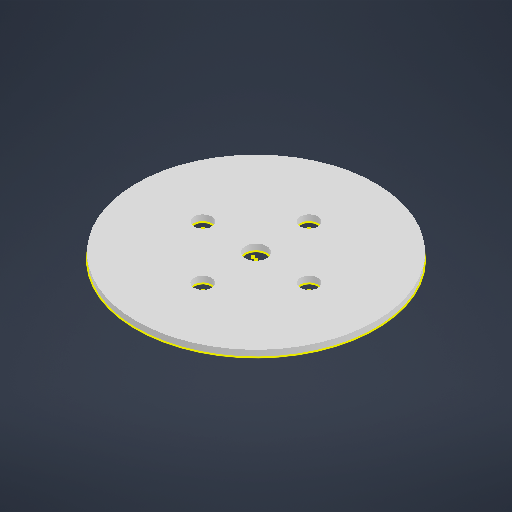
# Autodesk Inventor part: Part5
Saved by Autodesk Inventor 2025.2 (Build 292293000, 293)
## iProperties
Created: 2024-12-26
Part Number: Part5
Material: Generic
Document SubType Name: Sheet Metal
Designer: casey
Density: 1 g/cm^3
Appearance: Default
Flat Pattern Width: 5.715 cm
Flat Pattern Length: 5.715 cm
Flat Pattern Area: 32.6612 cm^2
Sheet Metal Rule: Default
Sheet Metal Width: 2.250 in
Sheet Metal Length: 2.250 in
Sheet Metal Area: 5.063 in^2
Author: casey
Autodesk Inventor part; units mm, degrees
ref_plane "YZ Plane" through (0, 0, 0) normal (1, 0, 0) x (0, 1, 0)
ref_plane "XZ Plane" through (0, 0, 0) normal (0, 1, 0) x (-1, 0, 0)
ref_plane "XY Plane" through (0, 0, 0) normal (0, 0, 1) x (1, 0, 0)
sketch "Sketch1" plane through (0, 0, 0) normal (0, 1, 0) x (-1, 0, 0)
  circle A0 centre (-0.8799, 12.92) radius 2.1
  circle A1 centre (-13.5799, 0.22) radius 2.1
  circle A2 centre (-0.8799, -12.48) radius 2.1
  circle A3 centre (11.8201, 0.22) radius 2.1
  circle A4 centre (-0.8799, 0.22) radius 28.575
  line L0 (-13.5799, 0.22) -> (-0.8799, 0.22)
  circle A5 centre (-0.8799, 0.22) radius 2.54
  point P0 (0, 0)
  dimension "d0" = 57.15
  dimension "d1" = 5.08
  constraints: 6 centre point, 2 end point, 1 coincident
  measures "d0" diameter of A4
  measures "d1" diameter of A5
extrude "Extrusion1" add sketch "Sketch1" along normal blind 1.5875
sketch "Sketch2" plane through (0, 0, 0) normal (0, 1, 0) x (-1, 0, 0)
  circle A0 centre (-0.8799, 0.22) radius 28.575 projected
  circle A1 centre (-13.5799, 0.22) radius 2.1 projected
  circle A2 centre (-0.8799, -12.48) radius 2.1 projected
  circle A3 centre (-0.8799, 0.22) radius 2.54 projected
  circle A4 centre (-0.8799, 12.92) radius 2.1 projected
  circle A5 centre (11.8201, 0.22) radius 2.1 projected
  point P0 (0, 0)
equation "\"BendRadius\" = Thickness"
equation "\"BendReliefWidth\" = Thickness"
equation "\"BendReliefDepth\" = 0.5 * Thickness"
equation "\"CornerReliefSize\" = 4 * Thickness"
equation "\"MinimumRemnant\" = 2 * Thickness"
equation "\"TransitionRadius\" = BendRadius"
equation "\"JacobiRadiusSize\" = BendRadius"
equation "\"GapSize\" = Thickness"
equation "\"Thickness\" = 1.5875"
body "Solid1"
